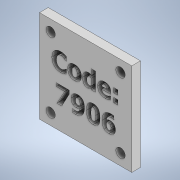
# Autodesk Inventor part: fireBoxSign
Saved by Autodesk Inventor 2021.2 (Build 252289000, 289)
## iProperties
Created: 2021-03-22
Part Number: fireBoxSign
Material: Generic
Document SubType Name: Modeling
Designer: robst
Density: 1 g/cm^3
Appearance: Default
Author: robst
Autodesk Inventor part; units mm, degrees
ref_plane "YZ Plane" through (0, 0, 0) normal (1, 0, 0) x (0, 1, 0)
ref_plane "XZ Plane" through (0, 0, 0) normal (0, 1, 0) x (-1, 0, 0)
ref_plane "XY Plane" through (0, 0, 0) normal (0, 0, 1) x (1, 0, 0)
sketch "Sketch2" plane through (0, 0, 0) normal (0, 0, 1) x (1, 0, 0)
  line L0 (-33.5407, -33.5407) -> (33.5407, -33.5407)
  line L1 (33.5407, -33.5407) -> (33.5407, 33.5407)
  line L2 (33.5407, 33.5407) -> (-33.5407, 33.5407)
  line L3 (-33.5407, 33.5407) -> (-33.5407, -33.5407)
  line L4 (-33.5407, -33.5407) -> (33.5407, 33.5407) construction
  line L5 (33.5407, -33.5407) -> (-33.5407, 33.5407) construction
  point P0 (0, 0)
  dimension "d6" = 67.0814
  dimension "d7" = 67.0814
  constraints: 12 end point, 2 midpoint, 2 parallel, 1 horizontal, 1 perpendicular
  measures "d6" distance of L1.end L2.end
  measures "d7" distance of L0.end L1.end
extrude "Extrusion2" add sketch "Sketch2" against normal blind 6.35
sketch "Sketch3" plane through (0, 0, 0) normal (0, 0, 1) x (1, 0, 0)
  line L0 (-25.4, -25.4) -> (25.4, -25.4) construction
  line L1 (25.4, -25.4) -> (25.4, 25.4) construction
  line L2 (25.4, 25.4) -> (-25.4, 25.4) construction
  line L3 (-25.4, 25.4) -> (-25.4, -25.4) construction
  line L4 (-25.4, -25.4) -> (25.4, 25.4) construction
  line L5 (25.4, -25.4) -> (-25.4, 25.4) construction
  point P0 (0, 0)
  dimension "d10" = 50.8
  dimension "d11" = 50.8
  constraints: 12 end point, 4 coincident, 2 midpoint, 2 parallel, 1 horizontal, 1 perpendicular
  measures "d10" distance of L1.end L2.end
  measures "d11" distance of L0.end L1.end
hole "Hole1" at (-25.4, 25.4, 0) at (25.4, 25.4, 0) at (25.4, -25.4, 0) at (-25.4, -25.4, 0) direction (0, 0, -1) diameter 6.7564 end through all clearance for "Socket Head Cap Screw" size "1/4" standard "Ansi Unified Screw Threads"
sketch "Sketch4" plane through (0, 0, 0) normal (0, 0, 1) x (1, 0, 0)
  line L0 (-22.225, -22.225) -> (22.225, -22.225) construction
  line L1 (22.225, -22.225) -> (22.225, 22.225) construction
  line L2 (22.225, 22.225) -> (-22.225, 22.225) construction
  line L3 (-22.225, 22.225) -> (-22.225, -22.225) construction
  line L4 (-22.225, -22.225) -> (22.225, 22.225) construction
  line L5 (22.225, -22.225) -> (-22.225, 22.225) construction
  line L6 (-22.225, 0) -> (22.225, 0) construction
  spline S0 degree 2 poles (-18.2781, 3.563) (-21.1392, 3.563) (-24.4943, 7.021) (-24.4943, 10.1497) knots 0 0 0 1 2 2 2
  spline S1 degree 2 poles (-24.4943, 10.1497) (-24.4943, 13.1652) (-21.1289, 16.757) (-18.2678, 16.757) knots 0 0 0 1 2 2 2
  spline S2 degree 2 poles (-18.2678, 16.757) (-17.5165, 16.757) (-16.3021, 16.582) (-15.7464, 16.438) knots 0 0 0 1 2 2 2
  spline S3 degree 2 poles (-15.7464, 16.438) (-15.3141, 16.3042) (-14.2952, 15.8616) (-13.9762, 15.697) knots 0 0 0 1 2 2 2
  line L7 (-13.9762, 15.697) -> (-13.9762, 12.6712)
  line L8 (-13.9762, 12.6712) -> (-14.2952, 12.6712)
  spline S4 degree 2 poles (-14.2952, 12.6712) (-14.5319, 12.877) (-15.2318, 13.4534) (-15.6743, 13.7209) knots 0 0 0 1 2 2 2
  spline S5 degree 2 poles (-15.6743, 13.7209) (-16.1169, 13.9988) (-17.1769, 14.3796) (-17.7635, 14.3796) knots 0 0 0 1 2 2 2
  spline S6 degree 2 poles (-17.7635, 14.3796) (-18.4531, 14.3796) (-19.5955, 13.9474) (-20.1203, 13.4019) knots 0 0 0 1 2 2 2
  spline S7 degree 2 poles (-20.1203, 13.4019) (-20.5938, 12.9182) (-21.201, 11.2612) (-21.201, 10.1394) knots 0 0 0 1 2 2 2
  spline S8 degree 2 poles (-21.201, 10.1394) (-21.201, 8.9559) (-20.5732, 7.3401) (-20.0586, 6.8461) knots 0 0 0 1 2 2 2
  spline S9 degree 2 poles (-20.0586, 6.8461) (-19.5646, 6.3624) (-18.3502, 5.9404) (-17.7429, 5.9404) knots 0 0 0 1 2 2 2
  spline S10 degree 2 poles (-17.7429, 5.9404) (-17.1152, 5.9404) (-15.9728, 6.3624) (-15.5817, 6.6196) knots 0 0 0 1 2 2 2
  spline S11 degree 2 poles (-15.5817, 6.6196) (-15.1494, 6.8769) (-14.5011, 7.4224) (-14.2643, 7.6385) knots 0 0 0 1 2 2 2
  line L9 (-14.2643, 7.6385) -> (-13.9762, 7.6385)
  line L10 (-13.9762, 7.6385) -> (-13.9762, 4.6539)
  spline S12 degree 2 poles (-13.9762, 4.6539) (-14.3261, 4.4893) (-15.2421, 4.0776) (-15.7361, 3.9335) knots 0 0 0 1 2 2 2
  spline S13 degree 2 poles (-15.7361, 3.9335) (-16.333, 3.7482) (-17.3724, 3.563) (-18.2781, 3.563) knots 0 0 0 1 2 2 2
  spline S14 degree 2 poles (-3.0772, 8.5957) (-3.0772, 6.2286) (-5.6605, 3.5115) (-8.0173, 3.5115) knots 0 0 0 1 2 2 2
  spline S15 degree 2 poles (-8.0173, 3.5115) (-10.3638, 3.5115) (-12.9676, 6.2286) (-12.9676, 8.5957) knots 0 0 0 1 2 2 2
  spline S16 degree 2 poles (-12.9676, 8.5957) (-12.9676, 10.9833) (-10.3638, 13.6901) (-8.0173, 13.6901) knots 0 0 0 1 2 2 2
  spline S17 degree 2 poles (-8.0173, 13.6901) (-5.6707, 13.6901) (-3.0772, 10.973) (-3.0772, 8.5957) knots 0 0 0 1 2 2 2
  spline S18 degree 2 poles (-6.1339, 8.5751) (-6.1339, 9.4293) (-6.4117, 10.5717) (-6.6588, 10.9113) knots 0 0 0 1 2 2 2
  spline S19 degree 2 poles (-6.6588, 10.9113) (-6.9263, 11.2715) (-7.5953, 11.5494) (-8.0173, 11.5494) knots 0 0 0 1 2 2 2
  spline S20 degree 2 poles (-8.0173, 11.5494) (-8.4289, 11.5494) (-9.0773, 11.3024) (-9.3449, 10.9525) knots 0 0 0 1 2 2 2
  spline S21 degree 2 poles (-9.3449, 10.9525) (-9.6022, 10.6231) (-9.9109, 9.4602) (-9.9109, 8.5751) knots 0 0 0 1 2 2 2
  spline S22 degree 2 poles (-9.9109, 8.5751) (-9.9109, 7.7003) (-9.6228, 6.6196) (-9.3861, 6.2903) knots 0 0 0 1 2 2 2
  spline S23 degree 2 poles (-9.3861, 6.2903) (-9.1494, 5.961) (-8.4289, 5.6522) (-7.9967, 5.6522) knots 0 0 0 1 2 2 2
  spline S24 degree 2 poles (-7.9967, 5.6522) (-7.6365, 5.6522) (-6.8955, 5.961) (-6.669, 6.2697) knots 0 0 0 1 2 2 2
  spline S25 degree 2 poles (-6.669, 6.2697) (-6.4117, 6.6299) (-6.1339, 7.6694) (-6.1339, 8.5751) knots 0 0 0 1 2 2 2
  line L11 (7.2145, 3.81) -> (4.2299, 3.81)
  line L12 (4.2299, 3.81) -> (4.2299, 4.8083)
  spline S26 degree 2 poles (4.2299, 4.8083) (3.9417, 4.5716) (3.2007, 4.0261) (2.9126, 3.882) knots 0 0 0 1 2 2 2
  spline S27 degree 2 poles (2.9126, 3.882) (2.5626, 3.7174) (1.8628, 3.5424) (1.3791, 3.5424) knots 0 0 0 1 2 2 2
  spline S28 degree 2 poles (1.3791, 3.5424) (-0.2573, 3.5424) (-2.1716, 6.2594) (-2.1716, 8.5236) knots 0 0 0 1 2 2 2
  spline S29 degree 2 poles (-2.1716, 8.5236) (-2.1716, 9.7792) (-1.5232, 11.6214) (-0.9571, 12.3007) knots 0 0 0 1 2 2 2
  spline S30 degree 2 poles (-0.9571, 12.3007) (-0.4323, 12.9285) (1.0498, 13.6489) (1.8731, 13.6489) knots 0 0 0 1 2 2 2
  spline S31 degree 2 poles (1.8731, 13.6489) (2.6244, 13.6489) (3.5918, 13.3299) (4.2299, 13.0005) knots 0 0 0 1 2 2 2
  line L13 (4.2299, 13.0005) -> (4.2299, 17.076)
  line L14 (4.2299, 17.076) -> (7.2145, 17.076)
  line L15 (7.2145, 17.076) -> (7.2145, 3.81)
  line L16 (4.2299, 6.4447) -> (4.2299, 11.148)
  spline S32 degree 2 poles (4.2299, 11.148) (4.0138, 11.2612) (3.2934, 11.4053) (3.0361, 11.4053) knots 0 0 0 1 2 2 2
  spline S33 degree 2 poles (3.0361, 11.4053) (1.9657, 11.4053) (0.8851, 9.9027) (0.8851, 8.5545) knots 0 0 0 1 2 2 2
  spline S34 degree 2 poles (0.8851, 8.5545) (0.8851, 7.1342) (1.7496, 5.8683) (2.7067, 5.8683) knots 0 0 0 1 2 2 2
  spline S35 degree 2 poles (2.7067, 5.8683) (3.0978, 5.8683) (3.9006, 6.1771) (4.2299, 6.4447) knots 0 0 0 1 2 2 2
  spline S36 degree 2 poles (14.4084, 3.5527) (11.6914, 3.5527) (8.7994, 6.1462) (8.7994, 8.5442) knots 0 0 0 1 2 2 2
  spline S37 degree 2 poles (8.7994, 8.5442) (8.7994, 10.8907) (11.4959, 13.6901) (13.9247, 13.6901) knots 0 0 0 1 2 2 2
  spline S38 degree 2 poles (13.9247, 13.6901) (16.1169, 13.6901) (18.3399, 11.3127) (18.3399, 9.1102) knots 0 0 0 1 2 2 2
  line L17 (18.3399, 9.1102) -> (18.3399, 8.0296)
  line L18 (18.3399, 8.0296) -> (11.784, 8.0296)
  spline S39 degree 2 poles (11.784, 8.0296) (11.8252, 7.3606) (12.3089, 6.4756) (12.7, 6.208) knots 0 0 0 1 2 2 2
  spline S40 degree 2 poles (12.7, 6.208) (13.0808, 5.9404) (14.11, 5.714) (14.7172, 5.714) knots 0 0 0 1 2 2 2
  spline S41 degree 2 poles (14.7172, 5.714) (15.2318, 5.714) (16.2404, 5.9404) (16.6623, 6.1359) knots 0 0 0 1 2 2 2
  spline S42 degree 2 poles (16.6623, 6.1359) (17.0328, 6.2903) (17.6503, 6.6711) (17.8459, 6.8152) knots 0 0 0 1 2 2 2
  line L19 (17.8459, 6.8152) -> (18.1649, 6.8152)
  line L20 (18.1649, 6.8152) -> (18.1649, 4.3452)
  spline S43 degree 2 poles (18.1649, 4.3452) (17.7944, 4.2011) (17.1975, 3.9541) (16.6623, 3.8306) knots 0 0 0 1 2 2 2
  spline S44 degree 2 poles (16.6623, 3.8306) (16.1786, 3.6968) (15.1494, 3.5527) (14.4084, 3.5527) knots 0 0 0 1 2 2 2
  spline S45 degree 2 poles (15.3964, 9.8307) (15.3759, 10.7775) (14.5422, 11.7758) (13.688, 11.7758) knots 0 0 0 1 2 2 2
  spline S46 degree 2 poles (13.688, 11.7758) (12.8132, 11.7758) (11.8252, 10.726) (11.7737, 9.8307) knots 0 0 0 1 2 2 2
  line L21 (11.7737, 9.8307) -> (15.3964, 9.8307)
  line L22 (23.4137, 3.81) -> (20.3982, 3.81)
  line L23 (20.3982, 3.81) -> (20.3982, 7.1651)
  line L24 (20.3982, 7.1651) -> (23.4137, 7.1651)
  line L25 (23.4137, 7.1651) -> (23.4137, 3.81)
  line L26 (23.4137, 10.0365) -> (20.3982, 10.0365)
  line L27 (20.3982, 10.0365) -> (20.3982, 13.3916)
  line L28 (20.3982, 13.3916) -> (23.4137, 13.3916)
  line L29 (23.4137, 13.3916) -> (23.4137, 10.0365)
  line L30 (-11.9075, -6.9734) -> (-17.3313, -17.152)
  line L31 (-17.3313, -17.152) -> (-20.8716, -17.152)
  line L32 (-20.8716, -17.152) -> (-15.2009, -6.8499)
  line L33 (-15.2009, -6.8499) -> (-21.2524, -6.8499)
  line L34 (-21.2524, -6.8499) -> (-21.2524, -4.452)
  line L35 (-21.2524, -4.452) -> (-11.9075, -4.452)
  line L36 (-11.9075, -4.452) -> (-11.9075, -6.9734)
  spline S47 degree 2 poles (-0.8336, -10.0918) (-0.8336, -11.7076) (-1.5849, -14.4041) (-2.3774, -15.3715) knots 0 0 0 1 2 2 2
  spline S48 degree 2 poles (-2.3774, -15.3715) (-3.2007, -16.3492) (-5.6296, -17.399) (-7.3998, -17.399) knots 0 0 0 1 2 2 2
  spline S49 degree 2 poles (-7.3998, -17.399) (-7.9967, -17.399) (-9.2934, -17.2446) (-9.5096, -17.1828) knots 0 0 0 1 2 2 2
  line L37 (-9.5096, -17.1828) -> (-9.5096, -14.6922)
  line L38 (-9.5096, -14.6922) -> (-9.2626, -14.6922)
  spline S50 degree 2 poles (-9.2626, -14.6922) (-9.0259, -14.8157) (-8.1408, -15.0833) (-7.3689, -15.0833) knots 0 0 0 1 2 2 2
  spline S51 degree 2 poles (-7.3689, -15.0833) (-6.7411, -15.0833) (-5.5781, -14.754) (-5.1665, -14.3938) knots 0 0 0 1 2 2 2
  spline S52 degree 2 poles (-5.1665, -14.3938) (-4.7239, -14.013) (-4.1476, -12.8912) (-4.0447, -12.0473) knots 0 0 0 1 2 2 2
  spline S53 degree 2 poles (-4.0447, -12.0473) (-4.7239, -12.4692) (-5.8972, -12.9221) (-6.772, -12.9221) knots 0 0 0 1 2 2 2
  spline S54 degree 2 poles (-6.772, -12.9221) (-7.4203, -12.9221) (-8.6245, -12.5721) (-9.1185, -12.2016) knots 0 0 0 1 2 2 2
  spline S55 degree 2 poles (-9.1185, -12.2016) (-9.7771, -11.6974) (-10.549, -10.0815) (-10.549, -8.8054) knots 0 0 0 1 2 2 2
  spline S56 degree 2 poles (-10.549, -8.8054) (-10.549, -7.8071) (-9.8698, -6.1295) (-9.2523, -5.512) knots 0 0 0 1 2 2 2
  spline S57 degree 2 poles (-9.2523, -5.512) (-8.6348, -4.8945) (-6.844, -4.1947) (-5.7428, -4.1947) knots 0 0 0 1 2 2 2
  spline S58 degree 2 poles (-5.7428, -4.1947) (-4.6313, -4.1947) (-2.9126, -4.8122) (-2.2951, -5.4606) knots 0 0 0 1 2 2 2
  spline S59 degree 2 poles (-2.2951, -5.4606) (-1.5746, -6.181) (-0.8336, -8.4657) (-0.8336, -10.0918) knots 0 0 0 1 2 2 2
  spline S60 degree 2 poles (-3.9932, -9.6184) (-3.9932, -8.579) (-4.3431, -7.241) (-4.6622, -6.8705) knots 0 0 0 1 2 2 2
  spline S61 degree 2 poles (-4.6622, -6.8705) (-4.8783, -6.5927) (-5.434, -6.3559) (-5.7531, -6.3559) knots 0 0 0 1 2 2 2
  spline S62 degree 2 poles (-5.7531, -6.3559) (-6.0412, -6.3559) (-6.5764, -6.5824) (-6.8234, -6.8705) knots 0 0 0 1 2 2 2
  spline S63 degree 2 poles (-6.8234, -6.8705) (-7.0395, -7.1175) (-7.3483, -8.0747) (-7.3483, -8.6407) knots 0 0 0 1 2 2 2
  spline S64 degree 2 poles (-7.3483, -8.6407) (-7.3483, -9.2582) (-7.0293, -10.0507) (-6.7617, -10.2874) knots 0 0 0 1 2 2 2
  spline S65 degree 2 poles (-6.7617, -10.2874) (-6.4838, -10.5241) (-5.7942, -10.7093) (-5.362, -10.7093) knots 0 0 0 1 2 2 2
  spline S66 degree 2 poles (-5.362, -10.7093) (-5.0018, -10.7093) (-4.2505, -10.5138) (-4.0138, -10.4109) knots 0 0 0 1 2 2 2
  spline S67 degree 2 poles (-4.0138, -10.4109) (-4.0138, -10.3183) (-3.9932, -9.9683) (-3.9932, -9.6184) knots 0 0 0 1 2 2 2
  spline S68 degree 2 poles (10.4564, -10.802) (10.4564, -12.4486) (9.9315, -14.9187) (9.3449, -15.7523) knots 0 0 0 1 2 2 2
  spline S69 degree 2 poles (9.3449, -15.7523) (8.7686, -16.5756) (6.9058, -17.4196) (5.5678, -17.4196) knots 0 0 0 1 2 2 2
  spline S70 degree 2 poles (5.5678, -17.4196) (4.2196, -17.4196) (2.3671, -16.5756) (1.7805, -15.7317) knots 0 0 0 1 2 2 2
  spline S71 degree 2 poles (1.7805, -15.7317) (1.1938, -14.8981) (0.669, -12.4486) (0.669, -10.802) knots 0 0 0 1 2 2 2
  spline S72 degree 2 poles (0.669, -10.802) (0.669, -9.1141) (1.1938, -6.7264) (1.7908, -5.8619) knots 0 0 0 1 2 2 2
  spline S73 degree 2 poles (1.7908, -5.8619) (2.3877, -5.018) (4.2711, -4.1947) (5.5678, -4.1947) knots 0 0 0 1 2 2 2
  spline S74 degree 2 poles (5.5678, -4.1947) (6.9366, -4.1947) (8.7686, -5.0592) (9.3552, -5.9134) knots 0 0 0 1 2 2 2
  spline S75 degree 2 poles (9.3552, -5.9134) (9.9315, -6.747) (10.4564, -9.2068) (10.4564, -10.802) knots 0 0 0 1 2 2 2
  spline S76 degree 2 poles (7.2557, -10.802) (7.2557, -8.4452) (6.4838, -6.5412) (5.5678, -6.5412) knots 0 0 0 1 2 2 2
  spline S77 degree 2 poles (5.5678, -6.5412) (4.6519, -6.5412) (3.8697, -8.4452) (3.8697, -10.8123) knots 0 0 0 1 2 2 2
  spline S78 degree 2 poles (3.8697, -10.8123) (3.8697, -13.1382) (4.6519, -15.073) (5.5678, -15.073) knots 0 0 0 1 2 2 2
  spline S79 degree 2 poles (5.5678, -15.073) (6.4735, -15.073) (7.2557, -13.1382) (7.2557, -10.802) knots 0 0 0 1 2 2 2
  spline S80 degree 2 poles (21.6744, -12.8294) (21.6744, -14.8363) (19.1323, -17.4196) (16.9093, -17.4196) knots 0 0 0 1 2 2 2
  spline S81 degree 2 poles (16.9093, -17.4196) (15.7978, -17.4196) (14.0585, -16.7815) (13.4513, -16.1537) knots 0 0 0 1 2 2 2
  spline S82 degree 2 poles (13.4513, -16.1537) (12.7309, -15.423) (11.959, -13.1073) (11.959, -11.4915) knots 0 0 0 1 2 2 2
  spline S83 degree 2 poles (11.959, -11.4915) (11.959, -9.8243) (12.6794, -7.2307) (13.4925, -6.2324) knots 0 0 0 1 2 2 2
  spline S84 degree 2 poles (13.4925, -6.2324) (14.2643, -5.2856) (16.7755, -4.2153) (18.4942, -4.2153) knots 0 0 0 1 2 2 2
  spline S85 degree 2 poles (18.4942, -4.2153) (19.122, -4.2153) (20.3776, -4.3799) (20.6041, -4.4314) knots 0 0 0 1 2 2 2
  line L39 (20.6041, -4.4314) -> (20.6041, -6.922)
  line L40 (20.6041, -6.922) -> (20.3776, -6.922)
  spline S86 degree 2 poles (20.3776, -6.922) (20.1512, -6.8088) (19.122, -6.5309) (18.4634, -6.5309) knots 0 0 0 1 2 2 2
  spline S87 degree 2 poles (18.4634, -6.5309) (16.9711, -6.5309) (15.345, -8.1055) (15.1494, -9.567) knots 0 0 0 1 2 2 2
  spline S88 degree 2 poles (15.1494, -9.567) (15.7772, -9.1656) (17.0637, -8.6922) (17.8767, -8.6922) knots 0 0 0 1 2 2 2
  spline S89 degree 2 poles (17.8767, -8.6922) (18.5663, -8.6922) (19.7704, -9.0627) (20.2335, -9.4126) knots 0 0 0 1 2 2 2
  spline S90 degree 2 poles (20.2335, -9.4126) (20.8922, -9.9169) (21.6744, -11.5533) (21.6744, -12.8294) knots 0 0 0 1 2 2 2
  spline S91 degree 2 poles (17.9591, -14.7437) (18.2061, -14.435) (18.4737, -13.7145) (18.4737, -12.9838) knots 0 0 0 1 2 2 2
  spline S92 degree 2 poles (18.4737, -12.9838) (18.4737, -12.3663) (18.1649, -11.5636) (17.887, -11.3268) knots 0 0 0 1 2 2 2
  spline S93 degree 2 poles (17.887, -11.3268) (17.5989, -11.0798) (16.8887, -10.9049) (16.4874, -10.9049) knots 0 0 0 1 2 2 2
  spline S94 degree 2 poles (16.4874, -10.9049) (16.1477, -10.9049) (15.4479, -11.0798) (15.1391, -11.2033) knots 0 0 0 1 2 2 2
  spline S95 degree 2 poles (15.1391, -11.2033) (15.1391, -11.2857) (15.1186, -11.6768) (15.1186, -11.9752) knots 0 0 0 1 2 2 2
  spline S96 degree 2 poles (15.1186, -11.9752) (15.1186, -13.0764) (15.4994, -14.4041) (15.7978, -14.7437) knots 0 0 0 1 2 2 2
  spline S97 degree 2 poles (15.7978, -14.7437) (16.0139, -15.0216) (16.5903, -15.2583) (16.899, -15.2583) knots 0 0 0 1 2 2 2
  spline S98 degree 2 poles (16.899, -15.2583) (17.1563, -15.2583) (17.7532, -15.001) (17.9591, -14.7437) knots 0 0 0 1 2 2 2
  point P0 (0, 0)
  dimension "d19" = 44.45
  dimension "d20" = 44.45
  constraints: 14 end point, 4 midpoint, 2 horizontal, 2 parallel, 1 perpendicular
  measures "d19" distance of L1.end L2.end
  measures "d20" distance of L0.end L1.end
extrude "Extrusion3" cut sketch "Sketch4" against normal blind 4.2333
equation "\"d6\" = outerWidth"
equation "\"d7\" = outerHeight"
equation "\"d8\" = thickness"
equation "\"d10\" = centerWidthBoltHole"
equation "\"d11\" = centerHeightBoltHole"
equation "\"d19\" = textBoxWidth"
equation "\"d20\" = textBoxHeight"
equation "\"d21\" = textDepth"
equation "\"centerWidthBoltHole\" = 50.8"
equation "\"centerHeightBoltHole\" = 50.8"
equation "\"boltHoleClearance\" = 6.7564"
equation "\"thickness\" = 6.35"
equation "\"textHeight\" = 12.7"
equation "\"textDepth\" = 0.666667 * thickness"
equation "\"outerWidth\" = 67.0814"
equation "\"outerHeight\" = 67.0814"
equation "\"textBoxWidth\" = 44.45"
equation "\"textBoxHeight\" = 44.45"
body "Solid2"
